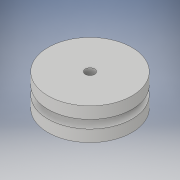
# Autodesk Inventor part: pulley wheel
Saved by Autodesk Inventor 2018 (Build 220112000, 112)
## iProperties
Created: 2018-11-15
Part Number: pulley wheel
Material: Generic
Document SubType Name: Modeling
Designer: Admin
Density: 1 g/cm^3
Appearance: Default
Author: Admin
Autodesk Inventor part; units mm, degrees
ref_plane "YZ Plane" through (0, 0, 0) normal (1, 0, 0) x (0, 1, 0)
ref_plane "XZ Plane" through (0, 0, 0) normal (0, 1, 0) x (-1, 0, 0)
ref_plane "XY Plane" through (0, 0, 0) normal (0, 0, 1) x (1, 0, 0)
sketch "Sketch1" plane through (0, 0, 0) normal (0, 0, 1) x (1, 0, 0)
  line L0 (0, 0) -> (27.94, 0)
  line L1 (27.94, 21.1836) -> (0, 21.1836)
  line L2 (0, 21.1836) -> (0, 0)
  circle A0 centre (27.94, 10.5918) radius 2.794
  line L3 (27.94, 0) -> (27.94, 7.7978)
  line L4 (27.94, 13.3858) -> (27.94, 21.1836)
  line L5 (27.94, 13.3858) -> (27.94, 7.7978) construction
  line L6 (0, 10.5918) -> (27.94, 10.5918) construction
  dimension "d0" = 27.94
  dimension "d1" = 21.1836
  dimension "d2" = 5.588
  constraints: 14 end point, 3 parallel, 3 point on circle, 2 horizontal, 2 line through centre, 2 perpendicular, 1 centre point, 1 collinear, 1 midpoint
  measures "d0" distance of L1.end L1.start
  measures "d1" distance of L1.start L0.end
  measures "d2" diameter of A0
revolve "Revolution1" add sketch "Sketch1" angle 360 about axis through (0, 21.1836, 0) along (0, -1, 0) contours L2 L1 L4 A0 L3 L0
sketch "Sketch2" plane through (0, 21.1836, 0) normal (0, 1, 0) x (1, 0, 0)
  circle A0 centre (0, 0) radius 3.175
  dimension "d4" = 6.35
  constraints: 1 centre point, 1 coincident
  measures "d4" diameter of A0
extrude "Extrusion1" cut sketch "Sketch2" against normal blind 25.4
body "Solid1"
